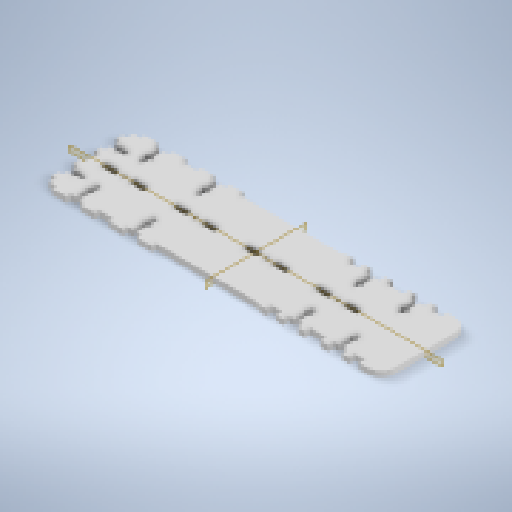
# Autodesk Inventor part: Крепление хвоста
Saved by Autodesk Inventor 2023.2 (Build 272271030, 271C)
## iProperties
Created: 2024-03-15
Part Number: Крепление хвоста
Material: Типовые
Document SubType Name: Modeling
Designer: I9232
Density: 1 g/cm^3
Appearance: По умолчанию
Author: I9232
Autodesk Inventor part; units mm, degrees
ref_plane "XZ Plane" through (0, 0, 0) normal (0, 1, 0) x (-1, 0, 0)
sketch "Эскиз1" plane through (0, 0, 0) normal (0, 1, 0) x (-1, 0, 0)
  line L0 (115.7159, 29.5) -> (-33.2841, 29.5)
  line L1 (-33.2841, -29.5) -> (115.7159, -29.5)
  line L2 (115.7159, -29.5) -> (115.7159, 29.5)
  line L3 (-33.2841, -29.5) -> (-33.2841, -30.9)
  line L4 (-119.2841, 30.9) -> (-119.2841, -30.9)
  line L5 (-33.2841, 29.5) -> (-33.2841, 30.9)
  line L6 (-166.2841, 0) -> (162.7159, 0) projected
  line L7 (-33.2841, 30.9) -> (-119.2841, 30.9)
  line L8 (-33.2841, -30.9) -> (-119.2841, -30.9)
  point P0 (0, 0)
  point P1 (115.7159, 0)
  point P2 (-119.2841, 0)
  dimension "d6" = 59
  dimension "d77" = 86
  dimension "d83" = 1.4
  constraints: 16 end point, 4 perpendicular, 2 equal length, 2 horizontal, 2 midpoint, 2 point on line, 2 vertical, 1 parallel
  measures "d6" distance of L1.end L0.start
  measures "d77" distance of L5.end L4.start
  measures "d83" distance of L0.end L5.end
extrude "Выдавливание1" add sketch "Эскиз1" along normal mid plane 4
fillet "Сопряжение1" radius 10 5 edges at (33.2841, 0, -29.5) (119.2841, 0, 30.9) (33.2841, 0, 29.5) (33.2841, 0, 30.9) (119.2841, 0, -30.9)
sketch "Эскиз2" plane through (0, -2, 0) normal (0, -1, 0) x (1, 0, 0)
  line L0 (-57.2159, -2) -> (-47.2159, -2) projected
  line L1 (-47.2159, 2) -> (-57.2159, 2) projected
  line L2 (-57.2159, -2) -> (-47.2159, -2) projected
  line L3 (-47.2159, 2) -> (-57.2159, 2) projected
  line L4 (-57.2159, -2) -> (-47.2159, -2) projected
  line L5 (-47.2159, 2) -> (-57.2159, 2) projected
  line L6 (-57.2159, -2) -> (-47.2159, -2) projected
  line L7 (-47.2159, 2) -> (-57.2159, 2) projected
  line L8 (42.7841, -2) -> (52.7841, -2) projected
  line L9 (52.7841, -2) -> (52.7841, 2) projected
  line L10 (52.7841, 2) -> (42.7841, 2) projected
  line L11 (42.7841, 2) -> (42.7841, -2) projected
  line L12 (62.7841, -2) -> (72.7841, -2) projected
  line L13 (72.7841, -2) -> (72.7841, 2) projected
  line L14 (72.7841, 2) -> (62.7841, 2) projected
  line L15 (62.7841, 2) -> (62.7841, -2) projected
  line L16 (12.7841, -2) -> (22.7841, -2) projected
  line L17 (22.7841, -2) -> (22.7841, 2) projected
  line L18 (22.7841, 2) -> (12.7841, 2) projected
  line L19 (12.7841, 2) -> (12.7841, -2) projected
  line L20 (-7.2159, -2) -> (2.7841, -2) projected
  line L21 (2.7841, -2) -> (2.7841, 2) projected
  line L22 (2.7841, 2) -> (-7.2159, 2) projected
  line L23 (-7.2159, 2) -> (-7.2159, -2) projected
  line L24 (-37.2159, -2) -> (-27.2159, -2) projected
  line L25 (-27.2159, -2) -> (-27.2159, 2) projected
  line L26 (-27.2159, 2) -> (-37.2159, 2) projected
  line L27 (-37.2159, 2) -> (-37.2159, -2) projected
  line L28 (-57.2159, -2) -> (-47.2159, -2) projected
  line L29 (-47.2159, -2) -> (-47.2159, 2) projected
  line L30 (-47.2159, 2) -> (-57.2159, 2) projected
  line L31 (-57.2159, 2) -> (-57.2159, -2) projected
  line L32 (-107.2159, -2) -> (-97.2159, -2) projected
  line L33 (-97.2159, -2) -> (-97.2159, 2) projected
  line L34 (-97.2159, 2) -> (-107.2159, 2) projected
  line L35 (-107.2159, 2) -> (-107.2159, -2) projected
  line L36 (-87.2159, -2) -> (-77.2159, -2) projected
  line L37 (-77.2159, -2) -> (-77.2159, 2) projected
  line L38 (-77.2159, 2) -> (-87.2159, 2) projected
  line L39 (-87.2159, 2) -> (-87.2159, -2) projected
  line L40 (-47.2159, -2) -> (-47.2159, 2) projected
  line L41 (-57.2159, 2) -> (-57.2159, -2) projected
  line L42 (-47.2159, -2) -> (-47.2159, 2) projected
  line L43 (-57.2159, 2) -> (-57.2159, -2) projected
  line L44 (-47.2159, -2) -> (-47.2159, 2) projected
  line L45 (-57.2159, 2) -> (-57.2159, -2) projected
  line L46 (-47.2159, -2) -> (-47.2159, 2) projected
  line L47 (-57.2159, 2) -> (-57.2159, -2) projected
  point P0 (0, 0)
extrude "Выдавливание2" cut sketch "Эскиз2" against normal up to surface (4 mm away)
sketch "Эскиз3" plane through (0, -2, 0) normal (0, -1, 0) x (1, 0, 0)
  circle A0 centre (57.7841, 0) radius 1.5
  circle A1 centre (7.7841, 0) radius 1.5
  circle A2 centre (-42.2159, 0) radius 1.5
  line L0 (62.7841, 2) -> (62.7841, -2)
  line L1 (62.7841, 0) -> (52.7841, 0) construction
  line L2 (52.7841, 2) -> (52.7841, -2)
  line L3 (12.7841, -2) -> (12.7841, 2)
  line L4 (12.7841, 0) -> (2.7841, 0) construction
  line L5 (2.7841, 2) -> (2.7841, -2)
  line L6 (-37.2159, -2) -> (-37.2159, 2)
  line L7 (-37.2159, 0) -> (-47.2159, 0) construction
  line L8 (-47.2159, 2) -> (-47.2159, -2)
  line L9 (-87.2159, -2) -> (-87.2159, 2)
  line L10 (-87.2159, 0) -> (-97.2159, 0) construction
  circle A3 centre (-92.2159, 0) radius 1.5
  point P0 (0, 0)
  point P1 (-92.2159, 0)
  dimension "d14" = 3
  constraints: 22 end point, 11 midpoint, 4 centre point, 4 coincident, 3 equal radius
  measures "d14" diameter of A0
extrude "Выдавливание3" cut sketch "Эскиз3" against normal up to surface (4 mm away)
sketch "Эскиз4" plane through (-115.7159, -2, 29.5) normal (-1, 0, 0) x (0, 0, 1)
  line L0 (-54.5, 4) -> (-49.5, 4)
  line L1 (-49.5, 4) -> (-49.5, 0)
  line L2 (-49.5, 0) -> (-54.5, 0)
  line L3 (-54.5, 0) -> (-54.5, 4)
  line L4 (-39.5, 4) -> (-34.5, 4)
  line L5 (-34.5, 4) -> (-34.5, 0)
  line L6 (-34.5, 0) -> (-39.5, 0)
  line L7 (-39.5, 0) -> (-39.5, 4)
  line L8 (-29.5, 0) -> (-29.5, 4)
  line L9 (-4.5, 4) -> (-9.5, 4)
  line L10 (-9.5, 4) -> (-9.5, 0)
  line L11 (-9.5, 0) -> (-4.5, 0)
  line L12 (-4.5, 0) -> (-4.5, 4)
  line L13 (-19.5, 4) -> (-24.5, 4)
  line L14 (-24.5, 4) -> (-24.5, 0)
  line L15 (-24.5, 0) -> (-19.5, 0)
  line L16 (-19.5, 0) -> (-19.5, 4)
  line L17 (-59, 4) -> (-59, 0) projected
  point P0 (-29.5, 2)
  dimension "d17" = 5
  dimension "d19" = 10
  dimension "d20" = 5
  dimension "d78" = 4.5
  constraints: 34 end point, 8 symmetric about line, 4 parallel, 2 horizontal, 2 perpendicular
  measures "d17" distance of L0.end L0.start
  measures "d19" distance between parallel lines of L7 L1
  measures "d20" distance of L5.end L6.end
  measures "d78" distance between parallel lines of L17 L3
sketch "Эскиз5" plane through (-115.7159, -2, -29.5) normal (0, 0, -1) x (-1, 0, 0)
  line L0 (0, 4) -> (-143.8971, 4) construction
  line L1 (-15, 4) -> (-5, 4)
  line L2 (-5, 4) -> (-5, 0)
  line L3 (-5, 0) -> (-15, 0)
  line L4 (-15, 0) -> (-15, 4)
  line L5 (0, 0) -> (-143.8971, 0) construction
  line L6 (-35, 4) -> (-25, 4)
  line L7 (-25, 4) -> (-25, 0)
  line L8 (-25, 0) -> (-35, 0)
  line L9 (-35, 0) -> (-35, 4)
  line L10 (0, 4) -> (0, 0) construction
  line L11 (-55, 4) -> (-45, 4)
  line L12 (-45, 4) -> (-45, 0)
  line L13 (-45, 0) -> (-55, 0)
  line L14 (-55, 0) -> (-55, 4)
  line L15 (-75, 4) -> (-65, 4)
  line L16 (-65, 4) -> (-65, 0)
  line L17 (-65, 0) -> (-75, 0)
  line L18 (-75, 0) -> (-75, 4)
  point P0 (-35, 0)
  point P1 (-225, 4)
  point P2 (-225, 0)
  dimension "d30" = 10
  dimension "d31" = 10
  dimension "d32" = 5
  dimension "d33" = 10
  dimension "d140" = 40
  constraints: 38 end point, 4 parallel, 4 point on line, 3 horizontal, 2 perpendicular, 16 other
  measures "d30" distance of L6.end L6.start
  measures "d31" distance of L1.end L1.start
  measures "d32" distance between parallel lines of L10 L2
  measures "d33" distance between parallel lines of L4 L7
  measures "d140" distance of L1.start L11.start
extrude "Выдавливание5" add sketch "Эскиз5" along normal blind 3
mirror "Зеркальное отражение1" about plane through (0, 0, 0) normal (0, 0, 1) of "Выдавливание5"
sketch "Эскиз7" plane through (0, -2, 0) normal (0, -1, 0) x (1, 0, 0)
  point P0 (0, 0)
sketch "Эскиз9" plane through (0, 2, 0) normal (0, 1, 0) x (1, 0, 0)
  line L0 (-97.1659, -29.5) -> (-94.2659, -29.5)
  line L1 (-94.2659, -14.6) -> (-97.1659, -14.6)
  line L2 (-165.2407, -29.5) -> (-26.1912, -29.5)
  line L3 (-92.9159, -21.4) -> (-92.9159, -19.6)
  line L4 (-98.5159, -19.6) -> (-98.5159, -21.4)
  line L5 (-95.7159, -14.6) -> (-95.7159, -29.5) construction
  line L6 (-97.1659, -14.6) -> (-97.1659, -19.6)
  line L7 (-97.1659, -21.4) -> (-97.1659, -29.5)
  line L8 (-98.5159, -21.4) -> (-97.1659, -21.4)
  line L9 (-94.2659, -21.4) -> (-92.9159, -21.4)
  line L10 (-92.9159, -19.6) -> (-94.2659, -19.6)
  line L11 (-97.1659, -19.6) -> (-98.5159, -19.6)
  line L12 (-94.2659, -29.5) -> (-94.2659, -21.4)
  line L13 (-94.2659, -19.6) -> (-94.2659, -14.6)
  line L14 (-57.1659, -19.6) -> (-58.5159, -19.6)
  line L15 (-57.1659, -14.6) -> (-57.1659, -19.6)
  line L16 (-54.2659, -19.6) -> (-54.2659, -14.6)
  line L17 (-54.2659, -14.6) -> (-57.1659, -14.6)
  line L18 (-58.5159, -21.4) -> (-57.1659, -21.4)
  line L19 (-58.5159, -19.6) -> (-58.5159, -21.4)
  line L20 (-52.9159, -21.4) -> (-52.9159, -19.6)
  line L21 (-54.2659, -21.4) -> (-52.9159, -21.4)
  line L22 (-55.7159, -14.6) -> (-55.7159, -29.5) construction
  line L23 (-57.1659, -21.4) -> (-57.1659, -29.5)
  line L24 (-54.2659, -29.5) -> (-54.2659, -21.4)
  line L25 (-57.1659, -29.5) -> (-54.2659, -29.5)
  line L26 (-52.9159, -19.6) -> (-54.2659, -19.6)
  line L27 (-89.9543, 0) -> (-81.423, 0) construction
  line L28 (-97.1659, 29.5) -> (-94.2659, 29.5)
  line L29 (-94.2659, 14.6) -> (-97.1659, 14.6)
  line L30 (-92.9159, 21.4) -> (-92.9159, 19.6)
  line L31 (-98.5159, 19.6) -> (-98.5159, 21.4)
  line L32 (-95.7159, 14.6) -> (-95.7159, 29.5) construction
  line L33 (-97.1659, 14.6) -> (-97.1659, 19.6)
  line L34 (-97.1659, 21.4) -> (-97.1659, 29.5)
  line L35 (-98.5159, 21.4) -> (-97.1659, 21.4)
  line L36 (-94.2659, 21.4) -> (-92.9159, 21.4)
  line L37 (-92.9159, 19.6) -> (-94.2659, 19.6)
  line L38 (-97.1659, 19.6) -> (-98.5159, 19.6)
  line L39 (-94.2659, 29.5) -> (-94.2659, 21.4)
  line L40 (-94.2659, 19.6) -> (-94.2659, 14.6)
  line L41 (-57.1659, 19.6) -> (-58.5159, 19.6)
  line L42 (-57.1659, 14.6) -> (-57.1659, 19.6)
  line L43 (-54.2659, 19.6) -> (-54.2659, 14.6)
  line L44 (-54.2659, 14.6) -> (-57.1659, 14.6)
  line L45 (-58.5159, 21.4) -> (-57.1659, 21.4)
  line L46 (-58.5159, 19.6) -> (-58.5159, 21.4)
  line L47 (-52.9159, 21.4) -> (-52.9159, 19.6)
  line L48 (-54.2659, 21.4) -> (-52.9159, 21.4)
  line L49 (-55.7159, 14.6) -> (-55.7159, 29.5) construction
  line L50 (-57.1659, 21.4) -> (-57.1659, 29.5)
  line L51 (-54.2659, 29.5) -> (-54.2659, 21.4)
  line L52 (-57.1659, 29.5) -> (-54.2659, 29.5)
  line L53 (-52.9159, 19.6) -> (-54.2659, 19.6)
  line L54 (-115.7159, 29.5) -> (-115.7159, -29.5) projected
  line L55 (-100.7159, -29.5) -> (-90.7159, -29.5) projected
  line L56 (-90.7159, 29.5) -> (-100.7159, 29.5) projected
  point P0 (0, 0)
  point P1 (-93.5909, -19.6)
  point P2 (-97.8409, -21.4)
  point P3 (-53.5909, -19.6)
  point P4 (-57.8409, -21.4)
  point P5 (-93.5909, 19.6)
  point P6 (-97.8409, 21.4)
  point P7 (-53.5909, 19.6)
  point P8 (-57.8409, 21.4)
  point P9 (-57.1659, -29.5)
  point P10 (-54.2659, -29.5)
  point P11 (-95.7159, -29.5)
  point P12 (-95.7159, 29.5)
  dimension "d48" = 2.9
  dimension "d49" = 1.8
  dimension "d50" = 5.6
  dimension "d52" = 1.35
  dimension "d58" = 40
  constraints: 108 end point, 32 symmetric about line, 10 parallel, 8 midpoint, 5 horizontal, 5 perpendicular, 2 coincident, 2 equal length, 29 other
  measures "d48" distance of L1.start L1.end
  measures "d49" distance of L4.start L4.end
  measures "d50" distance of L3.end L4.start
  measures "d52" distance of L6.end L4.start
  measures "d58" distance of point (-93.591, -19.6) point (-53.591, -19.6)
extrude "Выдавливание9" cut sketch "Эскиз9" against normal up to surface (4 mm away)
extrude "Выдавливание10" add sketch "Эскиз4" along normal blind 3
sketch "Эскиз12" plane through (109.2841, 2, -30.9) normal (0, 0, -1) x (-1, 0, 0)
  line L0 (70.9973, -4) -> (70.9973, 0)
  line L1 (5.3949, 0) -> (5.3949, -4)
  line L2 (0, 0) -> (76, 0) projected
  line L3 (5.3949, 0) -> (70.9973, 0)
  line L4 (76, -4) -> (0, -4) projected
  line L5 (70.9973, -4) -> (5.3949, -4)
  point P0 (109.2841, -2)
  point P1 (72.7517, 0)
  point P2 (72.7517, -4)
  constraints: 8 end point, 4 point on line
ref_plane "РабПлоскость1" through (-21.4617, -110.6568, -26.9) normal (0, 0, 1) x (1, -0.0000011, 0)
extrude "Выдавливание12" cut sketch "Эскиз12" against normal up to surface (4 mm away)
mirror "Зеркальное отражение2" about plane through (0, 0, 0) normal (0, 0, 1) of "Выдавливание12"
sketch "Эскиз13" plane through (103.8891, 2, -26.9) normal (0, 0, -1) x (-1, 0, 0)
  line L0 (65.6024, -4) -> (0, -4)
  line L1 (0, 0) -> (67.6024, 0)
  line L2 (22, 0) -> (27, 0)
  line L3 (27, 0) -> (27, -4)
  line L4 (27, -4) -> (22, -4)
  line L5 (22, -4) -> (22, 0)
  line L6 (7, 0) -> (12, 0)
  line L7 (12, 0) -> (12, -4)
  line L8 (12, -4) -> (7, -4)
  line L9 (7, -4) -> (7, 0)
  line L10 (0, -4) -> (0, 0) projected
  line L11 (41.1051, 0) -> (31.1051, 0) projected
  line L12 (0, 0) -> (0, -4) projected
  line L13 (32.8012, -2) -> (32.8012, -4) construction
  line L14 (65.6024, -4) -> (0, -4) projected
  line L15 (32.8012, -2) -> (32.8012, 0) construction
  line L16 (43.6024, 0) -> (38.6024, 0)
  line L17 (38.6024, 0) -> (38.6024, -4)
  line L18 (38.6024, -4) -> (43.6024, -4)
  line L19 (43.6024, -4) -> (43.6024, 0)
  line L20 (58.6024, 0) -> (53.6024, 0)
  line L21 (53.6024, 0) -> (53.6024, -4)
  line L22 (53.6024, -4) -> (58.6024, -4)
  line L23 (58.6024, -4) -> (58.6024, 0)
  point P0 (103.8891, -2)
  point P1 (7, -2)
  point P2 (58.6024, -2)
  point P3 (58.6024, 0)
  point P4 (53.6024, 0)
  point P5 (43.6024, 0)
  point P6 (38.6024, 0)
  point P7 (22, -4)
  point P8 (27, -4)
  point P9 (30, 0)
  point P10 (7, -4)
  point P11 (15, 0)
  point P12 (27, 0)
  point P13 (12, 0)
  dimension "d87" = 10
  dimension "d88" = 5
  dimension "d89" = 5
  dimension "d90" = 7
  constraints: 40 end point, 9 symmetric about line, 5 point on line, 4 parallel, 3 horizontal, 2 midpoint, 2 perpendicular, 1 collinear
  measures "d87" distance between parallel lines of L5 L7
  measures "d88" distance of L6.end L6.start
  measures "d89" distance of L2.end L2.start
  measures "d90" distance from line of point (7, -2) L10
ref_plane "РабПлоскость2" through (-21.4617, -110.6568, -30.9) normal (0, 0, -1) x (0.0000011, 1, 0)
extrude "Выдавливание13" add sketch "Эскиз13" along normal up to surface (4 mm away) contours L0 L21 L1 L23 | L0 L17 L1 L19 | L0 L5 L1 L3 | L0 L9 L1 L7
mirror "Зеркальное отражение3" about plane through (0, 0, 0) normal (0, 0, 1) of "Выдавливание13"
sketch "Эскиз14" plane through (0, 2, 0) normal (0, 1, 0) x (1, 0, 0)
  line L0 (56.7367, 26.9) -> (53.8367, 26.9)
  line L1 (53.8367, 14) -> (56.7367, 14)
  line L2 (52.4867, 17) -> (52.4867, 18.8)
  line L3 (58.0867, 18.8) -> (58.0867, 17)
  line L4 (55.2867, 14) -> (55.2867, 26.9) construction
  line L5 (56.7367, 14) -> (56.7367, 17)
  line L6 (56.7367, 18.8) -> (56.7367, 26.9)
  line L7 (58.0867, 17) -> (56.7367, 17)
  line L8 (53.8367, 17) -> (52.4867, 17)
  line L9 (52.4867, 18.8) -> (53.8367, 18.8)
  line L10 (56.7367, 18.8) -> (58.0867, 18.8)
  line L11 (53.8367, 26.9) -> (53.8367, 18.8)
  line L12 (53.8367, 17) -> (53.8367, 14)
  line L13 (60.2867, 26.9) -> (50.2867, 26.9) projected
  line L14 (91.8891, 26.9) -> (81.8891, 26.9) projected
  line L15 (45.2867, 26.9) -> (38.2867, 26.9) projected
  line L16 (88.3391, 26.9) -> (85.4391, 26.9)
  line L17 (85.4391, 14) -> (88.3391, 14)
  line L18 (84.0891, 17) -> (84.0891, 18.8)
  line L19 (89.6891, 18.8) -> (89.6891, 17)
  line L20 (86.8891, 14) -> (86.8891, 26.9) construction
  line L21 (88.3391, 14) -> (88.3391, 17)
  line L22 (88.3391, 18.8) -> (88.3391, 26.9)
  line L23 (89.6891, 17) -> (88.3391, 17)
  line L24 (85.4391, 17) -> (84.0891, 17)
  line L25 (84.0891, 18.8) -> (85.4391, 18.8)
  line L26 (88.3391, 18.8) -> (89.6891, 18.8)
  line L27 (85.4391, 26.9) -> (85.4391, 18.8)
  line L28 (85.4391, 17) -> (85.4391, 14)
  line L29 (71.453, 0) -> (50.2867, 0)
  line L30 (56.7367, -26.9) -> (53.8367, -26.9)
  line L31 (53.8367, -14) -> (56.7367, -14)
  line L32 (52.4867, -17) -> (52.4867, -18.8)
  line L33 (58.0867, -18.8) -> (58.0867, -17)
  line L34 (55.2867, -14) -> (55.2867, -26.9) construction
  line L35 (56.7367, -14) -> (56.7367, -17)
  line L36 (56.7367, -18.8) -> (56.7367, -26.9)
  line L37 (58.0867, -17) -> (56.7367, -17)
  line L38 (53.8367, -17) -> (52.4867, -17)
  line L39 (52.4867, -18.8) -> (53.8367, -18.8)
  line L40 (56.7367, -18.8) -> (58.0867, -18.8)
  line L41 (53.8367, -26.9) -> (53.8367, -18.8)
  line L42 (53.8367, -17) -> (53.8367, -14)
  line L43 (60.2867, -26.9) -> (50.2867, -26.9)
  line L44 (91.8891, -26.9) -> (81.8891, -26.9)
  line L45 (85.4391, -17) -> (85.4391, -14)
  line L46 (85.4391, -26.9) -> (85.4391, -18.8)
  line L47 (84.0891, -18.8) -> (85.4391, -18.8)
  line L48 (88.3391, -26.9) -> (85.4391, -26.9)
  line L49 (88.3391, -18.8) -> (88.3391, -26.9)
  line L50 (86.8891, -14) -> (86.8891, -26.9) construction
  line L51 (85.4391, -17) -> (84.0891, -17)
  line L52 (84.0891, -17) -> (84.0891, -18.8)
  line L53 (88.3391, -18.8) -> (89.6891, -18.8)
  line L54 (89.6891, -18.8) -> (89.6891, -17)
  line L55 (89.6891, -17) -> (88.3391, -17)
  line L56 (88.3391, -14) -> (88.3391, -17)
  line L57 (85.4391, -14) -> (88.3391, -14)
  point P0 (0, 0)
  point P1 (77.6159, 16.2969)
  point P2 (45.2867, -26.9)
  point P3 (77.6159, -16.2969)
  dimension "d93" = 5.6
  dimension "d94" = 1.8
  dimension "d95" = 2.9
  dimension "d96" = 1.35
  dimension "d97" = 2.9
  dimension "d98" = 8.1
  dimension "d99" = 3
  dimension "d100" = 5.6
  dimension "d101" = 1.8
  dimension "d102" = 2.9
  dimension "d103" = 1.35
  dimension "d104" = 2.9
  dimension "d105" = 8.1
  dimension "d106" = 3
  constraints: 110 end point, 34 symmetric about line, 20 parallel, 10 perpendicular, 7 horizontal, 6 midpoint, 4 equal length
  measures "d93" distance of L2.end L3.start
  measures "d94" distance of L2.start L2.end
  measures "d95" distance of L1.start L1.end
  measures "d96" distance of L8.start L2.start
  measures "d97" distance of L0.start L0.end
  measures "d98" distance of L0.end L9.end
  measures "d99" distance of L8.start L1.start
  measures "d100" distance of L25.start L26.end
  measures "d101" distance of L24.end L25.start
  measures "d102" distance of L28.end L21.start
  measures "d103" distance of L28.start L24.end
  measures "d104" distance of L16.start L27.start
  measures "d105" distance of L27.start L27.end
  measures "d106" distance of L28.start L28.end
extrude "Выдавливание14" cut sketch "Эскиз14" against normal up to surface (4 mm away)
sketch "Эскиз15" plane through (0, 2, 0) normal (0, 1, 0) x (1, 0, 0)
  line L0 (-105.4159, 16.45) -> (-105.4159, 13.55)
  line L1 (-115.7159, 13.55) -> (-115.7159, 16.45)
  line L2 (-105.4159, 15) -> (-115.7159, 15) construction
  line L3 (-110.4159, 17.8) -> (-112.2159, 17.8)
  line L4 (-112.2159, 12.2) -> (-110.4159, 12.2)
  line L5 (-115.7159, 16.45) -> (-112.2159, 16.45)
  line L6 (-110.4159, 16.45) -> (-105.4159, 16.45)
  line L7 (-110.4159, 12.2) -> (-110.4159, 13.55)
  line L8 (-110.4159, 16.45) -> (-110.4159, 17.8)
  line L9 (-112.2159, 17.8) -> (-112.2159, 16.45)
  line L10 (-112.2159, 13.55) -> (-112.2159, 12.2)
  line L11 (-105.4159, 13.55) -> (-110.4159, 13.55)
  line L12 (-112.2159, 13.55) -> (-115.7159, 13.55)
  line L13 (-115.7159, 20) -> (-115.7159, 10) projected
  line L14 (-105.4159, -13.55) -> (-105.4159, -16.45)
  line L15 (-115.7159, -16.45) -> (-115.7159, -13.55)
  line L16 (-105.4159, -15) -> (-115.7159, -15) construction
  line L17 (-110.4159, -12.2) -> (-112.2159, -12.2)
  line L18 (-112.2159, -17.8) -> (-110.4159, -17.8)
  line L19 (-115.7159, -13.55) -> (-112.2159, -13.55)
  line L20 (-110.4159, -13.55) -> (-105.4159, -13.55)
  line L21 (-110.4159, -17.8) -> (-110.4159, -16.45)
  line L22 (-110.4159, -13.55) -> (-110.4159, -12.2)
  line L23 (-112.2159, -12.2) -> (-112.2159, -13.55)
  line L24 (-112.2159, -16.45) -> (-112.2159, -17.8)
  line L25 (-105.4159, -16.45) -> (-110.4159, -16.45)
  line L26 (-112.2159, -16.45) -> (-115.7159, -16.45)
  line L27 (-115.7159, -10) -> (-115.7159, -20) projected
  point P0 (0, 0)
  dimension "d119" = 2.9
  dimension "d120" = 1.8
  dimension "d121" = 5.6
  dimension "d122" = 5
  dimension "d123" = 3.5
  dimension "d124" = 2.9
  dimension "d125" = 1.8
  dimension "d126" = 5.6
  dimension "d127" = 5
  dimension "d128" = 3.5
  constraints: 52 end point, 20 parallel, 10 equal length, 8 perpendicular, 6 horizontal, 6 midpoint
  measures "d119" distance of L0.start L0.end
  measures "d120" distance of L4.start L4.end
  measures "d121" distance of L3.end L4.start
  measures "d122" distance of L0.end L7.end
  measures "d123" distance of L10.start L1.start
  measures "d124" distance of L14.start L25.start
  measures "d125" distance of L18.start L18.end
  measures "d126" distance of L17.end L18.start
  measures "d127" distance of L25.start L21.end
  measures "d128" distance of L24.start L26.end
extrude "Выдавливание15" cut sketch "Эскиз15" against normal up to surface (4 mm away)
